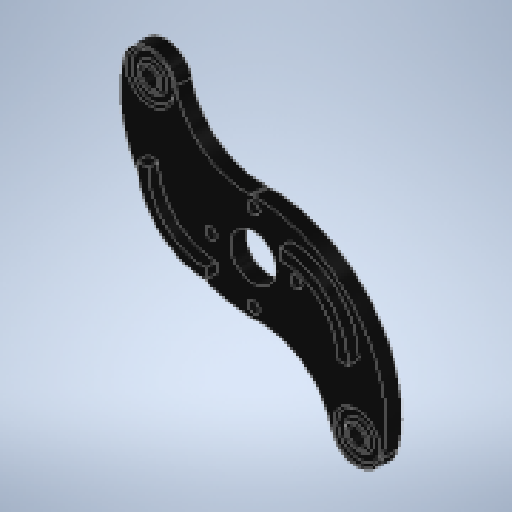
# Autodesk Inventor part: rotor_ver2
Saved by Autodesk Inventor 2024.3 (Build 283343010, 343A)
## iProperties
Created: 2025-06-26
Part Number: rotor_ver2
Material: アルミニウム 6061
Document SubType Name: Modeling
Designer: kshau
Density: 2.7 g/cm^3
Appearance: 光沢 - 黒
Author: kshau
Autodesk Inventor part; units mm, degrees
ref_plane "YZ Plane" through (0, 0, 0) normal (1, 0, 0) x (0, 1, 0)
ref_plane "XZ Plane" through (0, 0, 0) normal (0, 1, 0) x (-1, 0, 0)
ref_plane "XY Plane" through (0, 0, 0) normal (0, 0, 1) x (1, 0, 0)
sketch "スケッチ1" plane through (0, 0, 0) normal (0, 0, 1) x (1, 0, 0)
  circle A0 centre (0, 0) radius 27.5
  line L0 (0, 27.5) -> (0, 0)
  line L1 (8, 0) -> (19.445271, -19.445602)
  line L2 (0, 0) -> (27.5, 0)
  circle A1 centre (19.445271, -19.445602) radius 5
  circle A2 centre (0, 0) radius 10
  arc A3 (24.316088, -20.574825) -> (0, 10.000005) centre (0.018653, -14.941839) ccw
  line L3 (24.316088, -20.574825) -> (14.574455, -20.574825)
  arc A4 (14.574455, -20.574825) -> (0.517924, -9.986579) centre (1.227526, -23.669106) ccw
  arc A5 (-24.316088, 20.574825) -> (0, -10.000005) centre (-0.018653, 14.941839) ccw
  arc A6 (-14.574455, 20.574825) -> (-0.517924, 9.986579) centre (-1.227526, 23.669106) ccw
  circle A7 centre (-19.445271, 19.445602) radius 5
  point P0 (-0.517924, 9.986579)
  point P1 (0, -10)
  point P2 (0, 10.000005)
  dimension "d4" = 20
  dimension "d0" = 55
  dimension "d1" = 8
  dimension "d2" = 22.56381
  dimension "d3" = 10
  dimension "d5" = 9.74163
  dimension "d9" = 360
  constraints: 15 point on circle, 8 end point, 7 centre point, 3 coincident, 2 tangent, 1 horizontal, 1 parallel, 1 point on line, 1 vertical, 26 other
  measures "d0" diameter of A0
  measures "d1" distance from line of L0 L1.start
  measures "d2" distance of L1.start L1.end
  measures "d3" diameter of A1
  measures "d5" distance of L3.start L3.end
sketch "スケッチ1 outline for 押し出し1" plane through (0, 0, 0) normal (0, 0, 1) x (1, 0, 0)
  arc A0 (14.574455, -20.574825) -> (24.316088, -20.574825) centre (19.445271, -19.445602) ccw
  arc A1 (24.316088, -20.574825) -> (0, 10.000005) centre (0.018653, -14.941839) ccw
  arc A2 (0, 10) -> (-0.517924, 9.986579) centre (0, 0) ccw
  arc A3 (-0.517924, 9.986579) -> (-14.574455, 20.574825) centre (-1.227526, 23.669106) cw
  arc A4 (-14.574455, 20.574825) -> (-24.316088, 20.574825) centre (-19.445271, 19.445602) ccw
  arc A5 (-24.316088, 20.574825) -> (0, -10) centre (-0.018659, 14.941837) ccw
  arc A6 (0, -10) -> (0.517924, -9.986579) centre (0, 0) ccw
  arc A7 (0.517924, -9.986579) -> (14.574455, -20.574825) centre (1.227526, -23.669106) cw
extrude "押し出し1" add sketch "スケッチ1 outline for 押し出し1" along normal blind 3
sketch "スケッチ2" plane through (0, 0, 3) normal (0, 0, 1) x (1, 0, 0)
  circle A0 centre (0, 0) radius 4.25
  dimension "d13" = 8.5
  constraints: 1 centre point, 1 coincident
  measures "d13" diameter of A0
extrude "押し出し2" cut sketch "スケッチ2" against normal blind 3
sketch "スケッチ3" plane through (0, 0, 3) normal (0, 0, 1) x (1, 0, 0)
  arc A0 (-14.574455, 20.574825) -> (-24.316088, 20.574825) centre (-19.445271, 19.445602) ccw
  arc A1 (14.574455, -20.574825) -> (24.316088, -20.574825) centre (19.445271, -19.445602) ccw
  circle A2 centre (0, 0) radius 4.25
  point P0 (8, 0)
  point P1 (-8, 0)
  point P2 (0, 8)
  point P3 (-8, 0)
  point P4 (0, -8)
  dimension "d16" = 8
  dimension "d17" = 8
  dimension "d49" = 360
  constraints: 2 coincident, 5 other
  measures "d16" distance of A2.centre point (8, 0)
  measures "d17" distance of A2.centre point (-8, 0)
hole "穴1" at (-19.445271, 19.445602, 3) at (19.445271, -19.445602, 3) at (8, 0, 3) at (-8, 0, 3) at (0, 8, 3) at (0, -8, 3) direction (0, 0, -1) diameter 2.3 end through all
sketch "スケッチ4" plane through (0, 0, 3) normal (0, 0, 1) x (1, 0, 0)
  circle A0 centre (0, 0) radius 9.289
  circle A1 centre (8, 0) radius 1.15
  circle A2 centre (8, 0) radius 6.227
  circle A3 centre (0, 0) radius 8.107
  circle A4 centre (8, 0) radius 4.267399
  line L0 (6.969375, 6.141119) -> (6.969547, 4.141119)
  circle A5 centre (6.970301, -6.696881) radius 12.838
  circle A6 centre (0, 0) radius 20.909
  circle A7 centre (8, 0) radius 13.574
  line L1 (19.8083, -6.694589) -> (17.8083, -6.694761)
  arc A8 (17.8083, -6.694761) -> (6.969547, 4.141119) centre (6.970301, -6.696881) ccw
  circle A9 centre (-6.970301, 6.696881) radius 12.838
  line L2 (-19.8083, 6.694589) -> (-17.8083, 6.694761)
  arc A10 (-17.8083, 6.694761) -> (-6.969547, -4.141119) centre (-6.970301, 6.696881) ccw
  line L3 (-6.969375, -6.141119) -> (-6.969547, -4.141119)
  point P0 (6.969547, 4.141119)
  point P1 (-6.969547, -4.141119)
  dimension "d25" = 18.578
  dimension "d26" = 12.454
  dimension "d30" = 41.818
  dimension "d31" = 27.148
  dimension "d27" = 16.214
  dimension "d29" = 25.676
  dimension "d32" = 2
  dimension "d33" = 2
  dimension "d36" = 360
  constraints: 10 point on circle, 8 coincident, 8 end point, 5 centre point, 1 perpendicular, 38 other
  measures "d27" diameter of A3
  measures "d29" diameter of A5
  measures "d32" distance of L0.start L0.end
  measures "d33" distance of L1.start L1.end
extrude "押し出し3" add sketch "スケッチ4" along normal blind 2 contours A8 A4 A0 | A0 A4 A8 | A4 L0 A0 | A0 A5 A2 A8 A4 | A2 A5 L1 A8 | A9 L2 A10 A0 | A0 A10 L3 picked at (7.717949, 4.165451) picked at (9.179473, 4.022297)
sketch "スケッチ5" plane through (0, 0, 0) normal (0, 0, -1) x (-1, 0, 0)
  circle A0 centre (19.445271, 19.445602) radius 1.15
  circle A1 centre (-19.445271, -19.445602) radius 1.15
  point P0 (0, 0)
  constraints: 2 coincident
hole "穴2" at (-19.445271, 19.445602, 0) at (19.445271, -19.445602, 0) direction (0, 0, 1) diameter 3.2 end through all
sketch "スケッチ6" plane through (0, 0, 3) normal (0, 0, 1) x (1, 0, 0)
  circle A0 centre (-19.445271, 19.445602) radius 1.6
  circle A1 centre (-19.445271, 19.445602) radius 2.25
  circle A2 centre (-19.445271, 19.445602) radius 4
  circle A3 centre (19.445271, -19.445602) radius 1.6
  circle A4 centre (19.445271, -19.445602) radius 2.25
  circle A5 centre (19.445271, -19.445602) radius 4
  point P0 (0, 0)
  dimension "d51" = 4.5
  dimension "d52" = 8
  dimension "d53" = 4.5
  dimension "d54" = 8
  constraints: 4 centre point, 4 coincident
  measures "d51" diameter of A1
  measures "d52" diameter of A2
  measures "d53" diameter of A4
  measures "d54" diameter of A5
extrude "押し出し4" cut sketch "スケッチ6" against normal blind 0.5 contours A2 | A5
fillet "フィレット1" radius 0.5 4 edges at (-21.6953, 19.4456, 2.5) (17.1953, -19.4456, 2.5) (-23.4453, 19.4456, 3) (15.4453, -19.4456, 3)
